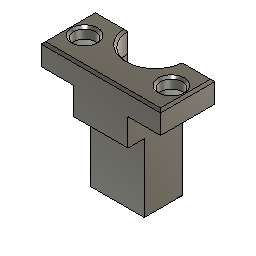
Wire_Protection_Final_x2 v3 (Autodesk Fusion 360 design; units mm, degrees)
Autodesk Fusion 360 part; units mm, degrees
sketch "Sketch1" plane through (0, 0, 0) normal (0, 0, 1) x (1, 0, 0)
  arc A0 (-5, 0) -> (5, 0) centre (0, 0) ccw
  line L0 (0, 0) -> (-5, 0) construction
  line L1 (0, 0) -> (5, 0) construction
  line L2 (-5, 0) -> (-11, 0)
  line L3 (-11, 0) -> (-11, -10)
  line L4 (-11, -10) -> (11, -10)
  line L5 (11, -10) -> (11, 0)
  line L6 (11, 0) -> (5, 0)
  dimension "d1" = 5
  dimension "d2" = 180
  dimension "d3" = 6
  dimension "d4" = 10
  dimension "d5" = 22
  constraint coincident A0.centre L0.start
  constraint parallel L0 L2
  constraint perpendicular L2 L3
  constraint perpendicular L3 L4
  constraint horizontal L2
  constraint perpendicular L4 L5
  constraint perpendicular L5 L6
  measures "d1" radius of A0
  measures "d2" angle of L0 L1
  measures "d3" distance of A0.start L2.end
  measures "d4" distance of L2.end L3.end
  measures "d5" distance of L3.end L4.end
extrude "Extrude1" add sketch "Sketch1" along normal blind 4
sketch "Sketch2" plane through (0, 0, 0) normal (0, 0, -1) x (1, 0, 0)
  line L0 (-11, 0) -> (-5, 0)
  arc A0 (5, 0) -> (-5, 0) centre (0, 0) ccw
  line L1 (5, 0) -> (11, 0)
  line L2 (11, 0) -> (11, 10)
  line L3 (11, 10) -> (-11, 10)
  line L4 (-11, 10) -> (-11, 0)
  line L5 (-5, 0) -> (-5, 10)
  line L6 (5, 10) -> (5, 0)
  dimension "d9" = 10
  constraint coincident L0.end A0.end
  constraint perpendicular L0 L5
  constraint coincident A0.start L1.start
  constraint coincident L3 L6.start
  measures "d9" distance of L5.end L6.start
extrude "Extrude2" add sketch "Sketch2" along normal blind 5 contours A0 L3 L5 L6
sketch "Sketch3" plane through (0, 0, -5) normal (0, 0, -1) x (1, 0, 0)
  line L0 (5, 10) -> (-5, 10)
  line L1 (-5, 10) -> (-5, 0)
  arc A0 (5, 0) -> (-5, 0) centre (0, 0) ccw
  line L2 (5, 0) -> (5, 10)
  line L3 (-5, 7) -> (5, 7)
  dimension "d12" = 7
  constraint coincident L1 L3.start
  constraint coincident L2 L3.end
  constraint perpendicular L2 L3
  measures "d12" distance of A0.start L3
extrude "Extrude3" add sketch "Sketch3" along normal blind 12.6 contours L1 A0 L2 L3
sketch "Sketch4" plane through (0, 0, 4) normal (0, 0, 1) x (-1, 0, 0)
  line L0 (5, 0) -> (11, 0)
  line L1 (11, 0) -> (11, 10)
  line L2 (11, 10) -> (-11, 10)
  line L3 (-11, 10) -> (-11, 0)
  line L4 (-11, 0) -> (-5, 0)
  arc A0 (5, 0) -> (-5, 0) centre (0, 0) ccw
  line L5 (11, 5) -> (-11, 5) construction
  line L6 (8, 0) -> (8, 5) construction
  line L7 (-8, 0) -> (-8, 5) construction
  constraint midpoint L1 L5.start
  constraint midpoint L3 L5.end
  constraint midpoint L0 L6.start
  constraint coincident L5 L6.end
  constraint perpendicular L5 L6
  constraint midpoint L4 L7.start
  constraint coincident L5 L7.end
  constraint perpendicular L5 L7
hole "Hole1" at (8, -5, 4) at (-8, -5, 4) direction (0, 0, -1) diameter 2.2 depth 4 tip angle 118 counterbore diameter 4 counterbore depth 2
sketch "Sketch5" plane through (0, 0, 2) normal (0, 0, 1) x (-1, 0, 0)
  circle A0 centre (8, 5) radius 2
  circle A1 centre (8, 5) radius 1.1
  point P0 (8, 5)
  constraint coincident P0 A0.centre
sketch "Sketch6" plane through (0, 0, 2) normal (0, 0, 1) x (-1, 0, 0)
  circle A0 centre (-8, 5) radius 2
  circle A1 centre (-8, 5) radius 1.1
  point P0 (-8, 5)
  constraint coincident P0 A0.centre
hole "Hole2" at (-8, -5, 2) at (8, -5, 2) direction (0, 0, -1) diameter 2.2 depth 8 tip angle 118 countersink diameter 4 countersink angle 130
chamfer "Chamfer1" distance 0.4 angle 45 8 edges at (11, -5, 4) (6.1353, -4.2768, 4) (0, -10, 4) (8, 0, 4) (0, -5, 4) (-9.8647, -4.2768, 4) (-8, 0, 4) (-11, -5, 4)
